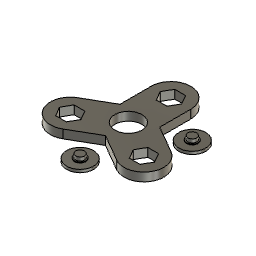
fidget spinner hex v2 (Autodesk Fusion 360 design; units mm, degrees)
Autodesk Fusion 360 part; units mm, degrees
sketch "Sketch1" plane through (0, 0, 0) normal (0, 0, 1) x (1, 0, 0)
  line L0 (-20, 20) -> (8, 20)
  line L1 (8, 20) -> (8, -10)
  line L2 (8, -10) -> (-20, -10)
  line L3 (-20, -10) -> (-20, 20)
  circle A0 centre (-6, -10) radius 14
  circle A1 centre (-6, 20) radius 14
  circle A2 centre (50, 15) radius 9.5
  circle A3 centre (50, 15) radius 4
  circle A4 centre (50, 15) radius 3.075
  circle A5 centre (-6, -10) radius 9.525
  line L4 (-13.5286, 20) -> (-9.7643, 13.48)
  line L5 (-9.7643, 13.48) -> (-2.2357, 13.48)
  line L6 (-2.2357, 13.48) -> (1.5286, 20)
  line L7 (1.5286, 20) -> (-2.2357, 26.52)
  line L8 (-2.2357, 26.52) -> (-9.7643, 26.52)
  line L9 (-9.7643, 26.52) -> (-13.5286, 20)
  point P0 (-6, 20)
  dimension "d1" = 28
  dimension "d2" = 30
  dimension "d3" = 28
  dimension "d4" = 28
  dimension "d5" = 19
  dimension "d6" = 8
  dimension "d7" = 6.15
  dimension "d8" = 19.05
  dimension "d9" = 13.04
  constraint horizontal L0
  constraint vertical L1
  constraint horizontal L2
  constraint vertical L3
  constraint midpoint L2 A0.centre
  constraint midpoint L0 P0
  constraint concentric A2 A3
  constraint concentric A2 A4
  constraint concentric A0 A5
  constraint coincident P0 A1.centre
  constraint coincident L0 L4.start
  measures "d1" distance of L0.start L0.end
  measures "d2" distance of L0.start L2.end
  measures "d3" diameter of A0
  measures "d4" diameter of A1
  measures "d5" diameter of A2
  measures "d6" diameter of A3
  measures "d7" diameter of A4
  measures "d8" diameter of A5
  measures "d9" distance of L5 L8
extrude "Extrude1" add sketch "Sketch1" along normal blind 6 contours L0 A1 L7 L8 L9 | L1 L3 A0 A1 | L0 A1 L4 L5 L6 | L2 A0 A5 | L2 A0 A5 makes body 1
extrude "Extrude2" add sketch "Sketch1" along normal blind 2 separate body contours A2 makes body 2
extrude "Extrude3" add sketch "Sketch1" along normal blind 2.5 contours A3 bodies 2
extrude "Extrude4" add sketch "Sketch1" along normal blind 5 contours A4 bodies 2
pattern_circular "C-Pattern1" count 3 over 360 about axis through (-6, -10, 0) along (0, 0, 1) of bodies 1 makes body 3 at (-19.6376, -26.997, 0) makes body 4 at (15.5386, -13.312, 0)
combine "Combine1" operation add target body 1 tool bodies 4 3
copy_body "CopyPasteBodies1" bodies 2 makes body 5
move_body "Move1" bodies 5 to x (1, 0, 0) y (0, 1, 0) z (0, 0, 1) at (12.2244, 20.8058, 8.5815)
move_body "Move2" bodies 5 to x (1, 0, 0) y (0, 1, 0) z (0, 0, 1) at (7.6363, -1.5808, -9.2172)
move_body "Move3" bodies 2 to x (1, 0, 0) y (0, 1, 0) z (0, 0, 1) at (-55, -65, 0)
move_body "Move4" bodies 5 to x (1, 0, 0) y (0, 1, 0) z (0, 0, 1) at (-40, -20, 0)
move_body "Move5" bodies 2 to x (1, 0, 0) y (0, 1, 0) z (0, 0, 1) at (0, 5, 0)
move_body "Move6" bodies 5 to x (1, 0, 0) y (0, 1, 0) z (0, 0, 1) at (-5, -10, 0)
move_body "Move7" bodies 5 to x (1, 0, 0) y (0, 1, 0) z (0, 0, 1) at (0, 2, 0)
move_body "Move8" bodies 5 to x (1, 0, 0) y (0, 1, 0) z (0, 0, 1) at (-2, 0, 0)
